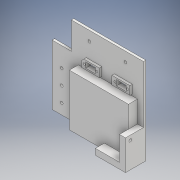
# Autodesk Inventor part: slot na baterie
Saved by Autodesk Inventor 2017 (Build 210142000, 142)
## iProperties
Created: 2019-08-28
Part Number: slot na baterie
Material: Ogólny
Document SubType Name: Modeling
Designer: patry
Density: 1 g/cm^3
Appearance: Gładki - biały
Author: patry
Autodesk Inventor part; units mm, degrees
ref_plane "YZ Plane" through (0, 0, 0) normal (1, 0, 0) x (0, 1, 0)
ref_plane "XZ Plane" through (0, 0, 0) normal (0, 1, 0) x (-1, 0, 0)
ref_plane "XY Plane" through (0, 0, 0) normal (0, 0, 1) x (1, 0, 0)
sketch "Szkic1" plane through (0, 0, 0) normal (0, 1, 0) x (-1, 0, 0)
  line L0 (44.7185, 35) -> (76.7185, 35)
  line L1 (76.7185, 35) -> (44.7185, 35)
  line L2 (44.7185, -65) -> (76.7185, -65)
  line L3 (76.7185, -65) -> (76.7185, 35)
  line L4 (44.7185, 80) -> (-75.2815, 80)
  line L5 (44.7185, 48) -> (44.7185, 80)
  line L6 (44.7185, -65) -> (44.7185, -55)
  line L7 (-75.2815, -65) -> (-75.2815, 48)
  line L8 (44.7185, -65) -> (-75.2815, -65)
  line L9 (-75.2815, 48) -> (-65.2815, 48)
  line L10 (-75.2815, 48) -> (-75.2815, 80)
  line L11 (44.7185, 35) -> (44.7185, -55)
  line L12 (-65.2815, -55) -> (44.7185, -55)
  line L13 (-65.2815, -55) -> (-65.2815, 48)
  line L14 (44.7185, 48) -> (-65.2815, 48)
  line L15 (44.7185, 35) -> (44.7185, 48)
  point P0 (0, 0)
  point P1 (14.7185, 64)
  point P2 (-45.2815, 64)
  point P3 (60.7185, 2.5)
  point P4 (60.7185, -47.5)
  point P5 (60.7185, -22.5)
  dimension "d2" = 32
  dimension "d3" = 45
  dimension "d4" = 32
  dimension "d5" = 32
  dimension "d23" = 100
  dimension "d24" = 10
  dimension "d25" = 10
  dimension "d26" = 120
  dimension "d27" = 16
  dimension "d28" = 16
  dimension "d29" = 50
  dimension "d30" = 16
  dimension "d31" = 16
  dimension "d32" = 60
  dimension "d33" = 17.5
  dimension "d34" = 30
  dimension "d126" = 42.5
  constraints: 32 end point, 7 perpendicular, 4 horizontal, 1 parallel, 1 vertical
  measures "d2" distance of L0.end L0.start
  measures "d3" distance of L4.start L0.start
  measures "d4" distance of L2.end L2.start
  measures "d5" distance of L7.end L4.end
  measures "d23" distance of L2.end L0.end
  measures "d24" distance of L2.start L6.end
  measures "d25" distance of L7.end L9.end
  measures "d26" distance of L4.start L4.end
  measures "d27" distance from line of L11 point (60.718, 2.5)
  measures "d28" distance from line of L11 point (60.718, -47.5)
  measures "d29" distance of point (60.718, 2.5) point (60.718, -47.5)
  measures "d30" distance from line of L14 point (14.718, 64)
  measures "d31" distance from line of L14 point (-45.282, 64)
  measures "d32" distance of point (-45.282, 64) point (14.718, 64)
  measures "d33" distance from line of L2 point (60.718, -47.5)
  measures "d34" distance from line of L10 point (-45.282, 64)
  measures "d126" distance from line of L2 point (60.718, -22.5)
extrude "Wyciągnięcie proste1" add sketch "Szkic1" along normal blind 4
extrude "Wyciągnięcie proste2" add sketch "Szkic1" against normal blind 15 contours L11 L12 L13 L14 L15
extrude "Wyciągnięcie proste3" add sketch "Szkic1" against normal blind 30 contours L6 L8 L7 L9 L13 L12
sketch "Szkic3" plane through (0, 4, 0) normal (0, 1, 0) x (1, 0, 0)
  line L0 (-76.7185, -35) -> (-44.7185, -35) projected
  line L1 (-44.7185, -35) -> (-44.7185, -80) projected
  line L2 (-44.7185, -80) -> (75.2815, -80) projected
  line L3 (75.2815, -80) -> (75.2815, 65) projected
  line L4 (75.2815, 65) -> (-76.7185, 65) projected
  line L5 (-76.7185, 65) -> (-76.7185, -35) projected
  line L6 (-44.7185, -48) -> (75.2815, -48) projected
  line L7 (-44.7185, 65) -> (-44.7185, -35) projected
  line L8 (-44.7185, 55) -> (65.2815, 55) projected
  line L9 (65.2815, 55) -> (65.2815, -48) projected
  line L10 (-29.7185, -17.5) -> (11.2815, -17.5)
  line L11 (11.2815, -17.5) -> (11.2815, 54.5)
  line L12 (11.2815, 54.5) -> (-29.7185, 54.5)
  line L13 (-29.7185, 54.5) -> (-29.7185, -17.5)
  line L14 (21.2815, -17.5) -> (62.2815, -17.5)
  line L15 (62.2815, -17.5) -> (62.2815, 54.5)
  line L16 (62.2815, 54.5) -> (21.2815, 54.5)
  line L17 (21.2815, 54.5) -> (21.2815, -17.5)
  line L18 (-16.7185, -35.5) -> (-0.7185, -35.5)
  line L19 (-0.7185, -35.5) -> (-0.7185, -26.5)
  line L20 (-0.7185, -26.5) -> (-16.7185, -26.5)
  line L21 (-16.7185, -26.5) -> (-16.7185, -35.5)
  line L22 (-16.7185, -35.5) -> (-0.7185, -26.5) construction
  line L23 (-0.7185, -35.5) -> (-16.7185, -26.5) construction
  circle A0 centre (-19.2185, -31) radius 1.75
  circle A1 centre (1.7815, -31) radius 1.75
  line L24 (-19.2185, -31) -> (1.7815, -31) construction
  circle A2 centre (52.7815, -31) radius 1.75
  line L25 (50.2815, -35.5) -> (50.2815, -26.5)
  line L26 (50.2815, -26.5) -> (34.2815, -26.5)
  line L27 (34.2815, -26.5) -> (34.2815, -35.5)
  line L28 (34.2815, -35.5) -> (50.2815, -26.5) construction
  line L29 (50.2815, -35.5) -> (34.2815, -26.5) construction
  line L30 (34.2815, -35.5) -> (50.2815, -35.5)
  line L31 (31.7815, -31) -> (52.7815, -31) construction
  circle A3 centre (31.7815, -31) radius 1.75
  point P0 (0, 0)
  point P1 (-8.7185, -31)
  point P2 (42.2815, -31)
  dimension "d35" = 41
  dimension "d36" = 72
  dimension "d37" = 41
  dimension "d38" = 72
  dimension "d39" = 10
  dimension "d40" = 15
  dimension "d41" = 30.5
  dimension "d50" = 30.5
  dimension "d78" = 16
  dimension "d79" = 9
  dimension "d80" = 3.5
  dimension "d81" = 3.5
  dimension "d82" = 10.5
  dimension "d83" = 10.5
  dimension "d86" = 4.5
  dimension "d87" = 4.5
  dimension "d88" = 20
  dimension "d89" = 9
  dimension "d90" = 16
  dimension "d91" = 9
  dimension "d92" = 3.5
  dimension "d93" = 3.5
  dimension "d94" = 10.5
  dimension "d95" = 10.5
  dimension "d96" = 4.5
  dimension "d97" = 4.5
  dimension "d102" = 9
  dimension "d127" = 20
  constraints: 44 end point, 8 parallel, 6 horizontal, 4 centre point, 4 coincident, 4 midpoint, 4 perpendicular
  measures "d35" distance of L12.end L11.end
  measures "d36" distance of L11.end L10.end
  measures "d37" distance of L15.end L16.end
  measures "d38" distance of L14.end L15.end
  measures "d39" distance between parallel lines of L11 L17
  measures "d40" distance between parallel lines of L7 L13
  measures "d41" distance between parallel lines of L6 L10
  measures "d50" distance between parallel lines of L6 L14
  measures "d78" distance of L20.end L19.end
  measures "d79" distance of L19.end L19.start
  measures "d80" diameter of A0
  measures "d81" diameter of A1
  measures "d82" distance of point (-8.718, -31) L24.start
  measures "d83" distance of point (-8.718, -31) L24.end
  measures "d86" distance from line of L18 L24.end
  measures "d87" distance from line of L18 L24.start
  measures "d88" distance from line of L11 point (-8.718, -31)
  measures "d89" distance between parallel lines of L10 L20
  measures "d90" distance of L26.end L25.end
  measures "d91" distance of L25.end L25.start
  measures "d92" diameter of A3
  measures "d93" diameter of A2
  measures "d94" distance of point (42.282, -31) L31.start
  measures "d95" distance of point (42.282, -31) L31.end
  measures "d96" distance from line of L30 L31.end
  measures "d97" distance from line of L30 L31.start
  measures "d102" distance between parallel lines of L14 L26
  measures "d127" distance from line of L15 point (42.282, -31)
extrude "Wyciągnięcie proste4" cut sketch "Szkic3" against normal blind 15 contours L13 L12 L11 L10 | L17 L16 L15 L14
extrude "Wyciągnięcie proste5" cut sketch "Szkic3" against normal blind 20 contours L21 L20 L19 L18 | A0 | A1 | A2 | L30 L27 L26 L25 | A3
sketch "Szkic4" plane through (0, -30, 0) normal (0, -1, 0) x (1, 0, 0)
  line L0 (-44.7185, 48) -> (-44.7185, -55) projected
  line L1 (-44.7185, -55) -> (65.2815, -55) projected
  line L2 (65.2815, -55) -> (65.2815, 48) projected
  line L3 (65.2815, 48) -> (-44.7185, 48) projected
  line L4 (-44.7185, -55) -> (-44.7185, -65) projected
  line L5 (-44.7185, -65) -> (75.2815, -65) projected
  line L6 (75.2815, -65) -> (75.2815, 48) projected
  line L7 (75.2815, 48) -> (65.2815, 48) projected
  line L8 (65.2815, 48) -> (65.2815, -55) projected
  line L9 (65.2815, -55) -> (-44.7185, -55) projected
  line L10 (65.2815, -55) -> (65.2815, 48) projected
  line L11 (75.2815, -65) -> (75.2815, 48) projected
  line L12 (65.2815, -15) -> (75.2815, -15)
  line L13 (75.2815, -15) -> (75.2815, 55)
  line L14 (75.2815, 55) -> (65.2815, 55)
  line L15 (65.2815, 55) -> (65.2815, -15)
  line L16 (-44.7185, -55) -> (65.2815, -55) projected
  line L17 (25.2815, -55) -> (-44.7185, -55)
  line L18 (-44.7185, -55) -> (-44.7185, -65)
  line L19 (-44.7185, -65) -> (25.2815, -65)
  line L20 (25.2815, -65) -> (25.2815, -55)
  dimension "d111" = 70
  dimension "d112" = 70
  dimension "d113" = 50
  dimension "d114" = 50
  constraints: 16 end point, 4 parallel, 4 point on line, 2 horizontal, 2 perpendicular
  measures "d111" distance between parallel lines of L14 L12
  measures "d112" distance between parallel lines of L18 L20
  measures "d113" distance between parallel lines of L5 L12
  measures "d114" distance between parallel lines of L20 L6
extrude "Wyciągnięcie proste6" cut sketch "Szkic4" against normal blind 15 contours L1 L20 L5 L4 | L7 L6 L12 L2 | L15 L14 L13 L7
hole "Otwór1" at (-14.7185, 0, 64) at (45.2815, 0, 64) at (-60.7185, 0, 2.5) at (-60.7185, 0, -47.5) at (-60.7185, 0, -22.5) direction (0, 1, 0) diameter 4.5 end through all clearance for "Śruba ze łbem płaskim obrobiona" size "M4" standard "ANSI Profil metryczny M"
sketch "Szkic5" plane through (0, -15, 0) normal (0, -1, 0) x (1, 0, 0)
  line L0 (-45, 48) -> (-10, 48)
  line L1 (65.2815, 48) -> (-44.7185, 48) projected
  line L2 (-45, 48) -> (-44.7185, 13.0011)
  line L3 (-44.7185, 13.0011) -> (-10, 48)
  point P0 (0, 0)
  dimension "d74" = 35
  constraints: 6 end point, 1 point on line
  measures "d74" distance of L0.start L2.end
extrude "Wyciągnięcie proste7" cut sketch "Szkic5" against normal blind 15
sketch "Szkic6" plane through (75.2815, 0, 80) normal (1, 0, 0) x (0, 0, -1)
  line L0 (145, -30) -> (145, 4) projected
  line L1 (145, -30) -> (95, -30) projected
  point P0 (80, 0)
  point P1 (102.5, -22)
  dimension "d117" = 42.5
  dimension "d118" = 8
  measures "d117" distance from line of L0 point (102.5, -22)
  measures "d118" distance from line of point (102.5, -22) L1
hole "Otwór2" at (75.2815, -22, -22.5) direction (-1, 0, 0) diameter 4.5 end through all clearance for "Śruba ze łbem płaskim obrobiona" size "M4" standard "ANSI Profil metryczny M"
sketch "Szkic8" plane through (0, -15, 0) normal (0, -1, 0) x (1, 0, 0)
  line L0 (-69, 21) -> (-69, 49)
  line L1 (-69, 49) -> (78, 49)
  line L2 (78, 49) -> (78, 21)
  line L3 (-33, -72) -> (-69, -72)
  line L4 (-69, -72) -> (-69, 21)
  line L5 (-33, 21) -> (-33, -72)
  line L6 (-33, 21) -> (78, 21)
  line L7 (11.2815, 17.5) -> (-29.7185, 17.5) projected
  line L8 (-29.7185, 17.5) -> (-29.7185, -54.5) projected
  line L9 (26.8332, 38) -> (56.6926, 38)
  line L10 (56.6926, 38) -> (56.6926, 24)
  line L11 (56.6926, 24) -> (26.8332, 24)
  line L12 (26.8332, 24) -> (26.8332, 38)
  line L13 (6, 38) -> (-24, 38)
  line L14 (-24, 38) -> (-24, 24)
  line L15 (-24, 24) -> (6, 24)
  line L16 (6, 24) -> (6, 38)
  line L17 (-29.7185, -54.5) -> (11.2815, -54.5) projected
  line L18 (21.2815, -54.5) -> (62.2815, -54.5) projected
  line L19 (62.2815, -54.5) -> (62.2815, 17.5) projected
  line L20 (62.2815, 17.5) -> (21.2815, 17.5) projected
  line L21 (65.2815, -55) -> (65.2815, -15) projected
  line L22 (78, 21) -> (65.2815, 21)
  line L23 (65.2815, 21) -> (65.2815, -15)
  line L24 (65.2815, -15) -> (78, -15)
  line L25 (78, -15) -> (78, 21)
  point P0 (0, 0)
  point P1 (65.2815, 48)
  constraints: 39 end point, 8 parallel, 5 horizontal, 4 perpendicular, 2 point on line
extrude "Wyciągnięcie proste9" cut sketch "Szkic8" against normal blind 15
sketch "Szkic9" plane through (0, -15, 0) normal (0, -1, 0) x (1, 0, 0)
  line L0 (-28, 43) -> (61, 43)
  line L1 (61, 43) -> (61, 22)
  line L2 (61, 22) -> (-28, 22)
  line L3 (-28, 22) -> (-28, 43)
  point P0 (0, 0)
  constraints: 8 end point, 2 parallel, 1 horizontal, 1 perpendicular
extrude "Wyciągnięcie proste10" cut sketch "Szkic9" against normal blind 11
equation "\"d4\" = d5"
equation "\"d24\" = d25"
equation "\"d27\" = 0.5 * d2"
equation "\"d28\" = d27"
equation "\"d30\" = d27"
equation "\"d31\" = d27"
equation "\"d37\" = d35"
equation "\"d38\" = d36"
equation "\"d50\" = d41"
equation "\"d80\" = d84"
equation "\"d81\" = d80"
equation "\"d82\" = d85"
equation "\"d83\" = d82"
equation "\"d92\" = d98"
equation "\"d93\" = d92"
equation "\"d94\" = d99"
equation "\"d95\" = d94"
equation "\"d102\" = d89"
equation "\"d84\" = 3.5"
equation "\"d98\" = 3.5"
equation "\"d85\" = 10.5"
equation "\"d99\" = 10.5"
